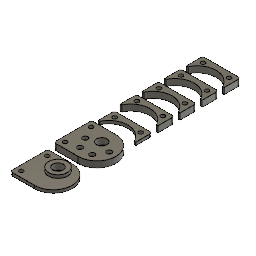
Z-axis Bosch POF1200 (Autodesk Fusion 360 design; units mm, degrees)
Autodesk Fusion 360 part; units mm, degrees
sketch "Sketch1" plane through (0, 0, 0) normal (0, 1, 0) x (1, 0, 0)
  line L0 (3, 0) -> (31, 0)
  line L1 (55, 24) -> (55, 24)
  line L2 (31, 48) -> (3, 48)
  line L3 (0, 45) -> (0, 3)
  arc A0 (55, 24) -> (31, 48) centre (31, 24) ccw
  arc A1 (31, 0) -> (55, 24) centre (31, 24) ccw
  arc A2 (0, 3) -> (3, 0) centre (3, 3) ccw
  arc A3 (3, 48) -> (0, 45) centre (3, 45) ccw
  circle A4 centre (7, 40.5) radius 2.6
  circle A5 centre (7, 7.5) radius 2.6
  circle A6 centre (30, 31) radius 6.5
  circle A7 centre (30, 31) radius 12
  circle A8 centre (15.3983, 25.8) radius 1.75
  circle A9 centre (22.3613, 12.3) radius 1.75
  circle A10 centre (37.6387, 12.3) radius 1.75
  circle A11 centre (44.531, 25.9) radius 1.75
  point P0 (55, 0)
  point P1 (0, 48)
  dimension "d1" = 55
  dimension "d2" = 48
  dimension "d3" = 24
  dimension "d4" = 24
  dimension "d5" = 3
  dimension "d6" = 3
  dimension "d7" = 5.2
  dimension "d8" = 5.2
  dimension "d9" = 7.5
  dimension "d10" = 7
  dimension "d11" = 7
  dimension "d12" = 7.5
  dimension "d13" = 13
  dimension "d14" = 30
  dimension "d15" = 17
  dimension "d16" = 24
  dimension "d17" = 3.5
  dimension "d18" = 3.5
  dimension "d19" = 3.5
  dimension "d20" = 3.5
  dimension "d21" = 24.5
  dimension "d23" = 13.5
  dimension "d79" = 15.5
  dimension "d80" = 5.2
  dimension "d81" = 15.4
  dimension "d82" = 5.1
  dimension "d83" = 20.2
  dimension "d84" = 20.2
  dimension "d85" = 18.7
  dimension "d86" = 18.7
  measures "d1" distance of origin P0
  measures "d2" distance of origin P1
  measures "d3" radius of A0
  measures "d4" radius of A1
  measures "d5" radius of A2
  measures "d6" radius of A3
  measures "d7" diameter of A4
  measures "d8" diameter of A5
  measures "d9" distance of L0 A5.centre
  measures "d10" distance of L3 A5.centre
  measures "d11" distance of L3 A4.centre
  measures "d12" distance of L2 A4.centre
  measures "d13" diameter of A6
  measures "d14" distance of L3 A6.centre
  measures "d15" distance of L2 A6.centre
  measures "d16" diameter of A7
  measures "d17" diameter of A8
  measures "d18" diameter of A9
  measures "d19" diameter of A10
  measures "d20" diameter of A11
  measures "d79" distance of A6.centre A8.centre
  measures "d80" distance of A6.centre A8.centre
  measures "d81" distance of A6.centre A11.centre
  measures "d82" distance of A6.centre A11.centre
  measures "d83" distance of A6.centre A9.centre
  measures "d84" distance of A6.centre A10.centre
  measures "d85" distance of A6.centre A10.centre
  measures "d86" distance of A6.centre A9.centre
extrude "Extrude1" add sketch "Sketch1" along normal blind 5 contours L0 L2 L3 A0 A1 A2 A3 | A8 | A9 | A10 | A11 makes body 1
extrude "Extrude2" add sketch "Sketch1" along normal blind 8 contours A7 bodies 1
copy_body "CopyPasteBodies1" bodies 1 makes body 2
copy_body "CopyPasteBodies2" bodies 1 makes body 3
move_body "Move1" bodies 3 to x (1, 0, 0) y (0, 1, 0) z (0, 0, 1) at (0, 0, -79.4684)
move_face "OffsetFaces1" offset 3 1 faces at (22.072, 5, -88.5782) on bodies 3
copy_body "CopyPasteBodies3" bodies 3 makes body 4
move_body "Move2" bodies 4 to x (1, 0, 0) y (0, 1, 0) z (0, 0, 1) at (0, 0, -70)
sketch "Sketch2" plane through (0, 8, 0) normal (0, 1, 0) x (-1, 0, 0)
  arc A0 (-3, -197.4684) -> (0, -194.4684) centre (-3, -194.4684) ccw
  line L0 (0, -194.4684) -> (0, -152.4684)
  arc A1 (0, -152.4684) -> (-3, -149.4684) centre (-3, -152.4684) ccw
  line L1 (-3, -149.4684) -> (-31, -149.4684)
  arc A2 (-31, -149.4684) -> (-31, -197.4684) centre (-31, -173.4684) ccw
  line L2 (-31, -197.4684) -> (-3, -197.4684)
  circle A3 centre (-7, -189.9684) radius 2.6
  circle A4 centre (-7, -156.9684) radius 2.6
  circle A5 centre (-30, -180.4684) radius 6.5
  circle A6 centre (-31, -173.4684) radius 24
extrude "Extrude3" cut sketch "Sketch2" against normal blind 8 contours A2 A6 bodies 4
sketch "Sketch3" plane through (0, 8, 0) normal (0, 1, 0) x (-1, 0, 0)
  arc A0 (-31, -197.4684) -> (-31, -149.4684) centre (-31, -173.4684) ccw
  line L0 (-31, -197.4684) -> (-3, -197.4684)
  arc A1 (-3, -197.4684) -> (0, -194.4684) centre (-3, -194.4684) ccw
  line L1 (0, -194.4684) -> (0, -152.4684)
  arc A2 (0, -152.4684) -> (-3, -149.4684) centre (-3, -152.4684) ccw
  line L2 (-3, -149.4684) -> (-31, -149.4684)
  circle A3 centre (-7, -189.9684) radius 2.6
  circle A4 centre (-7, -156.9684) radius 2.6
  line L3 (-20.7468, -197.4684) -> (-20.7468, -195.168)
  line L4 (-20.7468, -151.7688) -> (-20.7468, -149.4684)
extrude "Extrude4" cut sketch "Sketch3" against normal blind 10 contours A0 L2 L4 bodies 4
sketch "Sketch4" plane through (0, 8, 0) normal (0, 1, 0) x (-1, 0, 0)
  circle A0 centre (-7, -156.9684) radius 2.6
  circle A1 centre (-7, -189.9684) radius 2.6
  line L0 (-20.7468, -149.4684) -> (-20.7468, -151.7688)
  arc A2 (-31, -197.4684) -> (-20.7468, -151.7688) centre (-31, -173.4684) ccw
  line L1 (-31, -197.4684) -> (-3, -197.4684)
  arc A3 (-3, -197.4684) -> (0, -194.4684) centre (-3, -194.4684) ccw
  line L2 (0, -194.4684) -> (0, -152.4684)
  arc A4 (0, -152.4684) -> (-3, -149.4684) centre (-3, -152.4684) ccw
  line L3 (-3, -149.4684) -> (-20.7468, -149.4684)
  line L4 (-20.7468, -151.7688) -> (-20.7468, -202)
extrude "Extrude5" cut sketch "Sketch4" against normal blind 23 contours A2 L1 L4 bodies 4
copy_body "CopyPasteBodies4" bodies 4 makes body 5
move_body "Move3" bodies 5 to x (1, 0, 0) y (0, 1, 0) z (0, 0, 1) at (35, 0, 0)
copy_body "CopyPasteBodies5" bodies 4 5 makes body 6 makes body 7
move_body "Move4" bodies 6 7 to x (1, 0, 0) y (0, 1, 0) z (0, 0, 1) at (0, 0, -70)
move_body "Move5" bodies 6 1 2 3 5 7 4 to x (1, 0, 0) y (0, 1, 0) z (0, 0, 1) at (0, -8, 0)
move_body "Move12" bodies 7 5 4 6 3 to x (1, 0, 0) y (0, 1, 0) z (0, 0, 1) at (0, 0, 24)
move_face "MoveFace1" to x (1, 0, 0) y (0, 1, 0) z (0, 0, 1) at (0, 0, 14) 46 faces at (44.2186, -2.6667, -237.3241) (37.3333, 0, -219.4684) (42.4239, -2.6667, -223.9593) (55.7468, -2.6667, -197.002) (35, -2.6667, -226.4684) (35.5563, -2.6667, -242.2086) (43.9156, -5.3333, -195.4684) (49.8312, -2.6667, -243.4684) (37.3333, -8, -219.4684) (44.2186, -2.6667, -204.3241) (8.9156, -5.3333, -125.4684) (0, -2.6667, -156.4684) (20.7468, -5.3333, -172.7016) (35.5563, -2.6667, -172.2086) (44.2186, -2.6667, -167.3241) (55.7468, -2.6667, -127.002) (35, -2.6667, -156.4684) (44.2186, -2.6667, -134.3241) (37.3333, -8, -149.4684) (43.9156, -5.3333, -125.4684) (35.6418, -2.6667, -196.6139) (9.2186, -2.6667, -234.6127) (20.7468, -2.6667, -197.002) (20.7468, -5.3333, -242.7016) (0, -2.6667, -226.4684) (8.9156, -5.3333, -195.4684) (9.2186, -2.6667, -201.6127) (7.4239, -2.6667, -223.9593) (2.3333, -8, -219.4684) (0.6418, -2.6667, -196.6139) (2.3333, 0, -219.4684) (14.8312, -2.6667, -243.4684) (0.5563, -2.6667, -242.2086) (42.6613, -2.6667, -155.0634) (55.7468, -5.3333, -172.7016) (0.5563, -2.6667, -172.2086) (2.3333, 0, -149.4684) (20.7468, -2.6667, -127.002) (49.8312, -2.6667, -173.4684) (9.2186, -2.6667, -131.6127) (0.0136, -2.6667, -128.1832) (2.3333, -8, -149.4684) (14.8312, -2.6667, -173.4684) (7.6613, -2.6667, -155.0634) (37.3333, 0, -149.4684) (9.2186, -2.6667, -164.6127) on bodies 4 5 6 7
move_body "Move13" bodies 7 6 to x (1, 0, 0) y (0, 1, 0) z (0, 0, 1) at (0, 0, 14)
sketch "Sketch5" plane through (0, 0, 0) normal (0, 1, 0) x (-1, 0, 0)
  arc A0 (-3, -103.4684) -> (0, -100.4684) centre (-3, -100.4684) ccw
  line L0 (0, -100.4684) -> (0, -58.4684)
  arc A1 (0, -58.4684) -> (-3, -55.4684) centre (-3, -58.4684) ccw
  line L1 (-3, -55.4684) -> (-31, -55.4684)
  arc A2 (-31, -55.4684) -> (-31, -103.4684) centre (-31, -79.4684) ccw
  line L2 (-31, -103.4684) -> (-3, -103.4684)
  circle A3 centre (-7, -95.9684) radius 2.6
  circle A4 centre (-7, -62.9684) radius 2.6
  circle A5 centre (-30, -86.4684) radius 6.5
  circle A6 centre (-15.5, -79.9684) radius 3.25
  circle A7 centre (-22.5, -66.4684) radius 3.25
  circle A8 centre (-38, -66.4684) radius 3.25
  circle A9 centre (-46, -79.9684) radius 3.25
  circle A10 centre (-15.5, -79.9684) radius 1.75
  circle A11 centre (-22.5, -66.4684) radius 1.75
  circle A12 centre (-38, -66.4684) radius 1.75
  circle A13 centre (-46, -79.9684) radius 1.75
  dimension "d49" = 6.5
  dimension "d50" = 6.5
  dimension "d51" = 6.5
  dimension "d52" = 6.5
  dimension "d64" = 3.5
  dimension "d65" = 3.5
  dimension "d66" = 3.5
  dimension "d67" = 3.5
  measures "d49" diameter of A6
  measures "d50" diameter of A7
  measures "d51" diameter of A8
  measures "d52" diameter of A9
  measures "d64" diameter of A10
  measures "d65" diameter of A11
  measures "d66" diameter of A12
  measures "d67" diameter of A13
extrude "Extrude6" cut sketch "Sketch5" against normal blind 4 contours A6 | A10 bodies 3
extrude "Extrude7" cut sketch "Sketch5" against normal blind 4 contours A7 | A11 bodies 3
extrude "Extrude8" cut sketch "Sketch5" against normal blind 4 contours A8 | A12 bodies 3
extrude "Extrude9" cut sketch "Sketch5" against normal blind 4 contours A9 | A13 bodies 3
move_body "Move14" bodies 5 7 to x (1, 0, 0) y (0, 1, 0) z (0, 0, 1) at (-7, 0, 0)
extrude "Extrude10" cut sketch "Sketch5" against normal blind 9 contours A10 | A11 | A12 | A13 bodies 3
copy_body "CopyPasteBodies6" bodies 4 7 5 6 makes body 8 makes body 9 makes body 10 makes body 11
copy_body "CopyPasteBodies9" bodies 6 11 makes body 12 makes body 13
move_body "Move20" bodies 12 13 to x (1, 0, 0) y (0, 1, 0) z (0, 0, 1) at (0, 0, -56)
extrude "Extrude13" cut 1 faces at (2.3333, 0, -247.4684) along direction (0, -1, 0) blind 4 on bodies 12 bodies 12 13
move_body "Move21" bodies 7 11 9 6 4 12 13 8 5 10 to x (0, 0, 1) y (0, 1, 0) z (-1, 0, 0) at (-111.4684, 0, -160.4684)
move_body "Move22" bodies 12 13 to x (1, 0, 0) y (0, 1, 0) z (0, 0, 1) at (-56, 0, -28)
move_body "Move23" bodies 6 7 12 11 9 13 to x (1, 0, 0) y (0, 1, 0) z (0, 0, 1) at (-56, 0, -56)
extrude "Extrude14" cut 1 faces at (22.072, -3, -9.1098) along direction (0, -1, 0) blind 1 on bodies 1 bodies 1 2
move_body "Move24" bodies 5 10 to x (1, 0, 0) y (0, 1, 0) z (0, 0, 1) at (0, 0, -142)
move_body "Move25" bodies 12 13 to x (1, 0, 0) y (0, 1, 0) z (0, 0, 1) at (0, 0, 112)
move_body "Move26" bodies 10 5 to x (1, 0, 0) y (0, 1, 0) z (0, 0, 1) at (0, 0, 30)
